Autodesk Fusion 360 part; units mm, degrees
(part 3 of 3)
  spline S15 degree 5 poles (18.7244, -28.2025) (18.739, -28.2245) (18.7673, -28.2688) (18.8075, -28.3365) (18.8568, -28.4292) (18.9125, -28.5485) (18.964, -28.6701) (19.013, -28.7931) (19.0606, -28.917) (19.1072, -29.0413) (19.1528, -29.1663) (19.1969, -29.2919) (19.2391, -29.4186) (19.2791, -29.5463) (19.317, -29.6751) (19.3529, -29.8048) (19.3872, -29.9353) (19.42, -30.0665) (19.4516, -30.1982) (19.482, -30.3304) (19.5111, -30.4632) (19.5389, -30.5965) (19.5653, -30.7304) (19.5903, -30.8649) (19.614, -31) (19.6363, -31.1356) (19.6574, -31.2716) (19.6772, -31.4082) (19.6959, -31.5451) (19.7135, -31.6825) (19.7298, -31.8203) (19.745, -31.9585) (19.7591, -32.0971) (19.772, -32.2361) (19.7837, -32.3755) (19.7943, -32.5153) (19.8038, -32.6554) (19.8122, -32.7958) (19.8195, -32.9366) (19.8258, -33.0777) (19.831, -33.2191) (19.8351, -33.3608) (19.8382, -33.5028) (19.8402, -33.6451) (19.8412, -33.7877) (19.8411, -33.9305) (19.84, -34.0736) (19.8379, -34.217) (19.8348, -34.3605) (19.8307, -34.5044) (19.8256, -34.6484) (19.8195, -34.7927) (19.8124, -34.9372) (19.8044, -35.0819) (19.7953, -35.2268) (19.7853, -35.3719) (19.7743, -35.5171) (19.7624, -35.6626) (19.7495, -35.8082) (19.7356, -35.954) (19.7208, -36.1) (19.7051, -36.2461) (19.6884, -36.3924) (19.6707, -36.5388) (19.6522, -36.6854) (19.6327, -36.832) (19.6123, -36.9788) (19.591, -37.1258) (19.5687, -37.2728) (19.5456, -37.4199) (19.5215, -37.5672) (19.5015, -37.6851) (19.4862, -37.7735) (19.4757, -37.8325) (19.4704, -37.862) knots 0 0 0 0 0 0 0.01428571 0.02857143 0.04285714 0.05714286 0.07142857 0.08571429 0.1 0.11428571 0.12857143 0.14285714 0.15714286 0.17142857 0.18571429 0.2 0.21428571 0.22857143 0.24285714 0.25714286 0.27142857 0.28571429 0.3 0.31428571 0.32857143 0.34285714 0.35714286 0.37142857 0.38571429 0.4 0.41428571 0.42857143 0.44285714 0.45714286 0.47142857 0.48571429 0.5 0.51428571 0.52857143 0.54285714 0.55714286 0.57142857 0.58571429 0.6 0.61428571 0.62857143 0.64285714 0.65714286 0.67142857 0.68571429 0.7 0.71428571 0.72857143 0.74285714 0.75714286 0.77142857 0.78571429 0.8 0.81428571 0.82857143 0.84285714 0.85714286 0.87142857 0.88571429 0.9 0.91428571 0.92857143 0.94285714 0.95714286 0.97142857 0.98571429 1 1 1 1 1 1
  line L15 (18.7244, -28.2025) -> (16.4058, -24.7082)
  arc A30 (16.781, -22.5567) -> (16.4058, -24.7082) centre (17.7285, -23.8304) ccw
  arc A31 (16.781, -22.5567) -> (19.939, -19.8203) centre (0, 0) ccw
  arc A32 (22.1219, -19.7551) -> (19.939, -19.8203) centre (21.0648, -20.9395) ccw
  line L16 (22.1219, -19.7551) -> (25.2507, -22.5475)
  spline S16 degree 5 poles (25.2507, -22.5475) (25.2704, -22.565) (25.3102, -22.5993) (25.3715, -22.6488) (25.4563, -22.7108) (25.5664, -22.7829) (25.6794, -22.8512) (25.7942, -22.9172) (25.91, -22.9819) (26.0265, -23.0458) (26.1437, -23.1087) (26.2618, -23.1702) (26.3811, -23.23) (26.5018, -23.2878) (26.6239, -23.3436) (26.7472, -23.3976) (26.8715, -23.4501) (26.9967, -23.5013) (27.1226, -23.5513) (27.2492, -23.6001) (27.3764, -23.6479) (27.5044, -23.6944) (27.6332, -23.7396) (27.7628, -23.7835) (27.8931, -23.8261) (28.0241, -23.8675) (28.1558, -23.9077) (28.2881, -23.9468) (28.421, -23.9848) (28.5545, -24.0217) (28.6886, -24.0575) (28.8232, -24.0922) (28.9584, -24.1258) (29.0942, -24.1584) (29.2305, -24.1898) (29.3673, -24.2202) (29.5046, -24.2496) (29.6425, -24.2779) (29.7808, -24.3052) (29.9195, -24.3314) (30.0588, -24.3567) (30.1984, -24.3809) (30.3385, -24.4042) (30.4791, -24.4264) (30.6201, -24.4477) (30.7615, -24.468) (30.9033, -24.4873) (31.0454, -24.5056) (31.188, -24.523) (31.331, -24.5394) (31.4743, -24.5548) (31.6179, -24.5693) (31.762, -24.5829) (31.9063, -24.5955) (32.0511, -24.6071) (32.1961, -24.6179) (32.3415, -24.6277) (32.4871, -24.6365) (32.6331, -24.6445) (32.7794, -24.6515) (32.926, -24.6576) (33.0729, -24.6629) (33.22, -24.6672) (33.3674, -24.6705) (33.5151, -24.673) (33.6631, -24.6746) (33.8113, -24.6753) (33.9598, -24.6751) (34.1085, -24.674) (34.2574, -24.672) (34.4066, -24.6692) (34.5261, -24.6662) (34.6159, -24.6635) (34.6758, -24.6616) (34.7057, -24.6606) knots 0 0 0 0 0 0 0.01428571 0.02857143 0.04285714 0.05714286 0.07142857 0.08571429 0.1 0.11428571 0.12857143 0.14285714 0.15714286 0.17142857 0.18571429 0.2 0.21428571 0.22857143 0.24285714 0.25714286 0.27142857 0.28571429 0.3 0.31428571 0.32857143 0.34285714 0.35714286 0.37142857 0.38571429 0.4 0.41428571 0.42857143 0.44285714 0.45714286 0.47142857 0.48571429 0.5 0.51428571 0.52857143 0.54285714 0.55714286 0.57142857 0.58571429 0.6 0.61428571 0.62857143 0.64285714 0.65714286 0.67142857 0.68571429 0.7 0.71428571 0.72857143 0.74285714 0.75714286 0.77142857 0.78571429 0.8 0.81428571 0.82857143 0.84285714 0.85714286 0.87142857 0.88571429 0.9 0.91428571 0.92857143 0.94285714 0.95714286 0.97142857 0.98571429 1 1 1 1 1 1
  arc A33 (34.7057, -24.6606) -> (36.8493, -21.325) centre (0, 0) ccw
  spline S17 degree 5 poles (30.9994, -13.6023) (31.0235, -13.6129) (31.0713, -13.6348) (31.1418, -13.6701) (31.2334, -13.7214) (31.3447, -13.7916) (31.4538, -13.8661) (31.5615, -13.9431) (31.6685, -14.0216) (31.775, -14.101) (31.8808, -14.1814) (31.9859, -14.2633) (32.0898, -14.347) (32.1926, -14.4328) (32.2941, -14.5207) (32.3944, -14.6104) (32.4938, -14.7017) (32.5923, -14.7943) (32.6901, -14.888) (32.7871, -14.9829) (32.8834, -15.0788) (32.9789, -15.1759) (33.0735, -15.2743) (33.1673, -15.3739) (33.2602, -15.4747) (33.3523, -15.5767) (33.4436, -15.6798) (33.5341, -15.7839) (33.6239, -15.889) (33.7129, -15.9951) (33.8011, -16.1022) (33.8887, -16.2103) (33.9754, -16.3193) (34.0614, -16.4292) (34.1466, -16.5402) (34.2311, -16.652) (34.3149, -16.7647) (34.3979, -16.8783) (34.4801, -16.9928) (34.5617, -17.1081) (34.6425, -17.2243) (34.7226, -17.3412) (34.8019, -17.459) (34.8805, -17.5777) (34.9585, -17.6971) (35.0356, -17.8172) (35.1121, -17.9382) (35.1878, -18.0599) (35.2628, -18.1824) (35.3371, -18.3056) (35.4107, -18.4296) (35.4836, -18.5542) (35.5558, -18.6796) (35.6272, -18.8057) (35.6979, -18.9325) (35.7679, -19.06) (35.8372, -19.1881) (35.9058, -19.3169) (35.9737, -19.4464) (36.0409, -19.5766) (36.1073, -19.7074) (36.1731, -19.8388) (36.2381, -19.9709) (36.3025, -20.1036) (36.3661, -20.2369) (36.429, -20.3708) (36.4912, -20.5054) (36.5527, -20.6405) (36.6135, -20.7762) (36.6735, -20.9125) (36.7329, -21.0494) (36.7798, -21.1594) (36.8147, -21.2421) (36.8378, -21.2974) (36.8493, -21.325) knots 0 0 0 0 0 0 0.01428571 0.02857143 0.04285714 0.05714286 0.07142857 0.08571429 0.1 0.11428571 0.12857143 0.14285714 0.15714286 0.17142857 0.18571429 0.2 0.21428571 0.22857143 0.24285714 0.25714286 0.27142857 0.28571429 0.3 0.31428571 0.32857143 0.34285714 0.35714286 0.37142857 0.38571429 0.4 0.41428571 0.42857143 0.44285714 0.45714286 0.47142857 0.48571429 0.5 0.51428571 0.52857143 0.54285714 0.55714286 0.57142857 0.58571429 0.6 0.61428571 0.62857143 0.64285714 0.65714286 0.67142857 0.68571429 0.7 0.71428571 0.72857143 0.74285714 0.75714286 0.77142857 0.78571429 0.8 0.81428571 0.82857143 0.84285714 0.85714286 0.87142857 0.88571429 0.9 0.91428571 0.92857143 0.94285714 0.95714286 0.97142857 0.98571429 1 1 1 1 1 1
  line L17 (30.9994, -13.6023) -> (27.1596, -11.9162)
  arc A34 (26.3122, -9.9035) -> (27.1596, -11.9162) centre (27.7979, -10.4627) ccw
  arc A35 (26.3122, -9.9035) -> (27.4894, -5.8941) centre (0, 0) ccw
  arc A36 (29.2905, -4.6591) -> (27.4894, -5.8941) centre (29.0416, -6.2269) ccw
  line L18 (29.2905, -4.6591) -> (33.4323, -5.3166)
  spline S18 degree 5 poles (33.4323, -5.3166) (33.4583, -5.3207) (33.5104, -5.3281) (33.5887, -5.3365) (33.6936, -5.3428) (33.8252, -5.344) (33.9572, -5.3403) (34.0895, -5.3337) (34.2219, -5.3256) (34.3544, -5.3164) (34.4869, -5.3059) (34.6196, -5.2938) (34.7523, -5.2796) (34.8851, -5.263) (35.018, -5.2439) (35.1509, -5.2227) (35.2838, -5.1996) (35.4168, -5.175) (35.5497, -5.149) (35.6826, -5.1217) (35.8155, -5.093) (35.9483, -5.0629) (36.0811, -5.0314) (36.2138, -4.9983) (36.3465, -4.9637) (36.4791, -4.9277) (36.6117, -4.8903) (36.7441, -4.8516) (36.8765, -4.8117) (37.0087, -4.7706) (37.1408, -4.7282) (37.2729, -4.6847) (37.4048, -4.6398) (37.5366, -4.5938) (37.6683, -4.5466) (37.7998, -4.4982) (37.9312, -4.4486) (38.0624, -4.3979) (38.1935, -4.3461) (38.3245, -4.2932) (38.4553, -4.2392) (38.5859, -4.1841) (38.7163, -4.1279) (38.8466, -4.0706) (38.9767, -4.0123) (39.1066, -3.9529) (39.2363, -3.8924) (39.3658, -3.831) (39.4951, -3.7685) (39.6243, -3.705) (39.7532, -3.6406) (39.8819, -3.5751) (40.0104, -3.5086) (40.1386, -3.4412) (40.2667, -3.3727) (40.3945, -3.3033) (40.5221, -3.233) (40.6494, -3.1617) (40.7765, -3.0895) (40.9034, -3.0163) (41.03, -2.9422) (41.1564, -2.8672) (41.2825, -2.7912) (41.4084, -2.7144) (41.534, -2.6366) (41.6593, -2.558) (41.7844, -2.4784) (41.9092, -2.398) (42.0337, -2.3167) (42.1579, -2.2345) (42.2818, -2.1514) (42.3808, -2.0843) (42.4548, -2.0335) (42.5042, -1.9995) (42.5288, -1.9825) knots 0 0 0 0 0 0 0.01428571 0.02857143 0.04285714 0.05714286 0.07142857 0.08571429 0.1 0.11428571 0.12857143 0.14285714 0.15714286 0.17142857 0.18571429 0.2 0.21428571 0.22857143 0.24285714 0.25714286 0.27142857 0.28571429 0.3 0.31428571 0.32857143 0.34285714 0.35714286 0.37142857 0.38571429 0.4 0.41428571 0.42857143 0.44285714 0.45714286 0.47142857 0.48571429 0.5 0.51428571 0.52857143 0.54285714 0.55714286 0.57142857 0.58571429 0.6 0.61428571 0.62857143 0.64285714 0.65714286 0.67142857 0.68571429 0.7 0.71428571 0.72857143 0.74285714 0.75714286 0.77142857 0.78571429 0.8 0.81428571 0.82857143 0.84285714 0.85714286 0.87142857 0.88571429 0.9 0.91428571 0.92857143 0.94285714 0.95714286 0.97142857 0.98571429 1 1 1 1 1 1
  arc A37 (42.5288, -1.9825) -> (42.5288, 1.9825) centre (0, 0) ccw
  spline S19 degree 5 poles (33.4323, 5.3166) (33.4583, 5.3207) (33.5104, 5.3281) (33.5887, 5.3365) (33.6936, 5.3428) (33.8252, 5.344) (33.9572, 5.3403) (34.0895, 5.3337) (34.2219, 5.3256) (34.3544, 5.3164) (34.4869, 5.3059) (34.6196, 5.2938) (34.7523, 5.2796) (34.8851, 5.263) (35.018, 5.2439) (35.1509, 5.2227) (35.2838, 5.1996) (35.4168, 5.175) (35.5497, 5.149) (35.6826, 5.1217) (35.8155, 5.093) (35.9483, 5.0629) (36.0811, 5.0314) (36.2138, 4.9983) (36.3465, 4.9637) (36.4791, 4.9277) (36.6117, 4.8903) (36.7441, 4.8516) (36.8765, 4.8117) (37.0087, 4.7706) (37.1408, 4.7282) (37.2729, 4.6847) (37.4048, 4.6398) (37.5366, 4.5938) (37.6683, 4.5466) (37.7998, 4.4982) (37.9312, 4.4486) (38.0624, 4.3979) (38.1935, 4.3461) (38.3245, 4.2932) (38.4553, 4.2392) (38.5859, 4.1841) (38.7163, 4.1279) (38.8466, 4.0706) (38.9767, 4.0123) (39.1066, 3.9529) (39.2363, 3.8924) (39.3658, 3.831) (39.4951, 3.7685) (39.6243, 3.705) (39.7532, 3.6406) (39.8819, 3.5751) (40.0104, 3.5086) (40.1386, 3.4412) (40.2667, 3.3727) (40.3945, 3.3033) (40.5221, 3.233) (40.6494, 3.1617) (40.7765, 3.0895) (40.9034, 3.0163) (41.03, 2.9422) (41.1564, 2.8672) (41.2825, 2.7912) (41.4084, 2.7144) (41.534, 2.6366) (41.6593, 2.558) (41.7844, 2.4784) (41.9092, 2.398) (42.0337, 2.3167) (42.1579, 2.2345) (42.2818, 2.1514) (42.3808, 2.0843) (42.4548, 2.0335) (42.5042, 1.9995) (42.5288, 1.9825) knots 0 0 0 0 0 0 0.01428571 0.02857143 0.04285714 0.05714286 0.07142857 0.08571429 0.1 0.11428571 0.12857143 0.14285714 0.15714286 0.17142857 0.18571429 0.2 0.21428571 0.22857143 0.24285714 0.25714286 0.27142857 0.28571429 0.3 0.31428571 0.32857143 0.34285714 0.35714286 0.37142857 0.38571429 0.4 0.41428571 0.42857143 0.44285714 0.45714286 0.47142857 0.48571429 0.5 0.51428571 0.52857143 0.54285714 0.55714286 0.57142857 0.58571429 0.6 0.61428571 0.62857143 0.64285714 0.65714286 0.67142857 0.68571429 0.7 0.71428571 0.72857143 0.74285714 0.75714286 0.77142857 0.78571429 0.8 0.81428571 0.82857143 0.84285714 0.85714286 0.87142857 0.88571429 0.9 0.91428571 0.92857143 0.94285714 0.95714286 0.97142857 0.98571429 1 1 1 1 1 1
  line L19 (33.4323, 5.3166) -> (29.2905, 4.6591)
  arc A38 (27.4894, 5.8941) -> (29.2905, 4.6591) centre (29.0416, 6.2269) ccw
  arc A39 (27.4894, 5.8941) -> (26.3122, 9.9035) centre (0, 0) ccw
  arc A40 (27.1596, 11.9162) -> (26.3122, 9.9035) centre (27.7979, 10.4627) ccw
  line L20 (27.1596, 11.9162) -> (30.9994, 13.6023)
  spline S20 degree 5 poles (30.9994, 13.6023) (31.0235, 13.6129) (31.0713, 13.6348) (31.1418, 13.6701) (31.2334, 13.7214) (31.3447, 13.7916) (31.4538, 13.8661) (31.5615, 13.9431) (31.6685, 14.0216) (31.775, 14.101) (31.8808, 14.1814) (31.9859, 14.2633) (32.0898, 14.347) (32.1926, 14.4328) (32.2941, 14.5207) (32.3944, 14.6104) (32.4938, 14.7017) (32.5923, 14.7943) (32.6901, 14.888) (32.7871, 14.9829) (32.8834, 15.0788) (32.9789, 15.1759) (33.0735, 15.2743) (33.1673, 15.3739) (33.2602, 15.4747) (33.3523, 15.5767) (33.4436, 15.6798) (33.5341, 15.7839) (33.6239, 15.889) (33.7129, 15.9951) (33.8011, 16.1022) (33.8887, 16.2103) (33.9754, 16.3193) (34.0614, 16.4292) (34.1466, 16.5402) (34.2311, 16.652) (34.3149, 16.7647) (34.3979, 16.8783) (34.4801, 16.9928) (34.5617, 17.1081) (34.6425, 17.2243) (34.7226, 17.3412) (34.8019, 17.459) (34.8805, 17.5777) (34.9585, 17.6971) (35.0356, 17.8172) (35.1121, 17.9382) (35.1878, 18.0599) (35.2628, 18.1824) (35.3371, 18.3056) (35.4107, 18.4296) (35.4836, 18.5542) (35.5558, 18.6796) (35.6272, 18.8057) (35.6979, 18.9325) (35.7679, 19.06) (35.8372, 19.1881) (35.9058, 19.3169) (35.9737, 19.4464) (36.0409, 19.5766) (36.1073, 19.7074) (36.1731, 19.8388) (36.2381, 19.9709) (36.3025, 20.1036) (36.3661, 20.2369) (36.429, 20.3708) (36.4912, 20.5054) (36.5527, 20.6405) (36.6135, 20.7762) (36.6735, 20.9125) (36.7329, 21.0494) (36.7798, 21.1594) (36.8147, 21.2421) (36.8378, 21.2974) (36.8493, 21.325) knots 0 0 0 0 0 0 0.01428571 0.02857143 0.04285714 0.05714286 0.07142857 0.08571429 0.1 0.11428571 0.12857143 0.14285714 0.15714286 0.17142857 0.18571429 0.2 0.21428571 0.22857143 0.24285714 0.25714286 0.27142857 0.28571429 0.3 0.31428571 0.32857143 0.34285714 0.35714286 0.37142857 0.38571429 0.4 0.41428571 0.42857143 0.44285714 0.45714286 0.47142857 0.48571429 0.5 0.51428571 0.52857143 0.54285714 0.55714286 0.57142857 0.58571429 0.6 0.61428571 0.62857143 0.64285714 0.65714286 0.67142857 0.68571429 0.7 0.71428571 0.72857143 0.74285714 0.75714286 0.77142857 0.78571429 0.8 0.81428571 0.82857143 0.84285714 0.85714286 0.87142857 0.88571429 0.9 0.91428571 0.92857143 0.94285714 0.95714286 0.97142857 0.98571429 1 1 1 1 1 1
  arc A41 (36.8493, 21.325) -> (34.7057, 24.6606) centre (0, 0) ccw
  spline S21 degree 5 poles (25.2507, 22.5475) (25.2704, 22.565) (25.3102, 22.5993) (25.3715, 22.6488) (25.4563, 22.7108) (25.5664, 22.7829) (25.6794, 22.8512) (25.7942, 22.9172) (25.91, 22.9819) (26.0265, 23.0458) (26.1437, 23.1087) (26.2618, 23.1702) (26.3811, 23.23) (26.5018, 23.2878) (26.6239, 23.3436) (26.7472, 23.3976) (26.8715, 23.4501) (26.9967, 23.5013) (27.1226, 23.5513) (27.2492, 23.6001) (27.3764, 23.6479) (27.5044, 23.6944) (27.6332, 23.7396) (27.7628, 23.7835) (27.8931, 23.8261) (28.0241, 23.8675) (28.1558, 23.9077) (28.2881, 23.9468) (28.421, 23.9848) (28.5545, 24.0217) (28.6886, 24.0575) (28.8232, 24.0922) (28.9584, 24.1258) (29.0942, 24.1584) (29.2305, 24.1898) (29.3673, 24.2202) (29.5046, 24.2496) (29.6425, 24.2779) (29.7808, 24.3052) (29.9195, 24.3314) (30.0588, 24.3567) (30.1984, 24.3809) (30.3385, 24.4042) (30.4791, 24.4264) (30.6201, 24.4477) (30.7615, 24.468) (30.9033, 24.4873) (31.0454, 24.5056) (31.188, 24.523) (31.331, 24.5394) (31.4743, 24.5548) (31.6179, 24.5693) (31.762, 24.5829) (31.9063, 24.5955) (32.0511, 24.6071) (32.1961, 24.6179) (32.3415, 24.6277) (32.4871, 24.6365) (32.6331, 24.6445) (32.7794, 24.6515) (32.926, 24.6576) (33.0729, 24.6629) (33.22, 24.6672) (33.3674, 24.6705) (33.5151, 24.673) (33.6631, 24.6746) (33.8113, 24.6753) (33.9598, 24.6751) (34.1085, 24.674) (34.2574, 24.672) (34.4066, 24.6692) (34.5261, 24.6662) (34.6159, 24.6635) (34.6758, 24.6616) (34.7057, 24.6606) knots 0 0 0 0 0 0 0.01428571 0.02857143 0.04285714 0.05714286 0.07142857 0.08571429 0.1 0.11428571 0.12857143 0.14285714 0.15714286 0.17142857 0.18571429 0.2 0.21428571 0.22857143 0.24285714 0.25714286 0.27142857 0.28571429 0.3 0.31428571 0.32857143 0.34285714 0.35714286 0.37142857 0.38571429 0.4 0.41428571 0.42857143 0.44285714 0.45714286 0.47142857 0.48571429 0.5 0.51428571 0.52857143 0.54285714 0.55714286 0.57142857 0.58571429 0.6 0.61428571 0.62857143 0.64285714 0.65714286 0.67142857 0.68571429 0.7 0.71428571 0.72857143 0.74285714 0.75714286 0.77142857 0.78571429 0.8 0.81428571 0.82857143 0.84285714 0.85714286 0.87142857 0.88571429 0.9 0.91428571 0.92857143 0.94285714 0.95714286 0.97142857 0.98571429 1 1 1 1 1 1
  line L21 (25.2507, 22.5475) -> (22.1219, 19.7551)
  arc A42 (19.939, 19.8203) -> (22.1219, 19.7551) centre (21.0648, 20.9395) ccw
  arc A43 (19.939, 19.8203) -> (16.781, 22.5567) centre (0, 0) ccw
  line L22 (0, 0) -> (0, 15) construction
  circle A44 centre (0, 15) radius 3.5
  dimension "d12" = 7
  constraint coincident A1.centre A3.centre
  constraint vertical L22
  constraint coincident L22.end A44.centre
  measures "d12" diameter of A44
extrude "Extrude4" add sketch "Sketch2 (2)" along normal blind 5 contours A44 in component "Spur Gear (11 teeth)"
extrude "Extrude5" cut 1 faces at (-2.701, 14.3431, 0) along direction (0, 0, 1) blind 5 in component "Spur Gear (11 teeth)"
extrude "Extrude6" cut 1 faces at (0.7112, -13.871, -5) along direction (0, 0, 1) blind 5 in component "Spur Gear (11 teeth)"
component "Spur Gear (11 teeth)" placed x (1, 0, 0) y (0, 1, 0) z (0, 0, 1) at (0, 0, 0)
